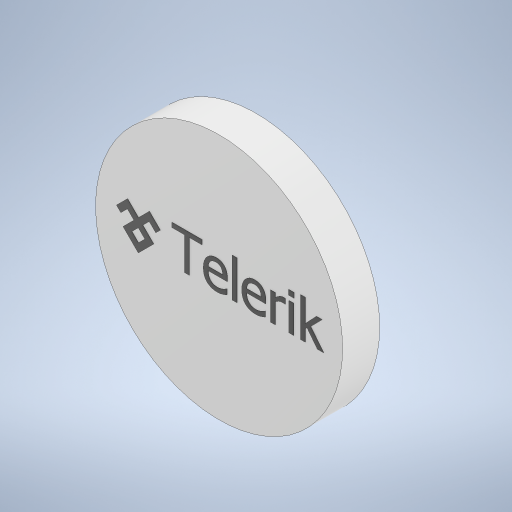
# Autodesk Inventor part: Logo Wheel
Saved by Autodesk Inventor 2023 (Build 270158000, 158)
## iProperties
Created: 2022-05-02
Part Number: Logo Wheel
Material: Phenolic Resin
Document SubType Name: Modeling
Designer: Devin
Density: 1.38 g/cm^3
Appearance: Smooth - White
Author: Devin
Autodesk Inventor part; units mm, degrees
ref_plane "YZ Plane" through (0, 0, 0) normal (1, 0, 0) x (0, 1, 0)
ref_plane "XZ Plane" through (0, 0, 0) normal (0, 1, 0) x (-1, 0, 0)
ref_plane "XY Plane" through (0, 0, 0) normal (0, 0, 1) x (1, 0, 0)
sketch "Sketch1" plane through (0, 0, 0) normal (0, 0, 1) x (1, 0, 0)
  circle A0 centre (0, 0) radius 10.16
  dimension "d0" = 20.32
  constraints: 1 centre point, 1 coincident
  measures "d0" diameter of A0
extrude "Extrusion1" add sketch "Sketch1" along normal blind 3.048
shell "Shell1" thickness 1.27 removed faces 1 at (6.5114, 0.3794, 0)
sketch "Sketch2" plane through (0, 0, 1.778) normal (0, 0, -1) x (-1, 0, 0)
  circle A0 centre (0, 0) radius 2.032
  circle A1 centre (0, 0) radius 0.635
  dimension "d4" = 4.064
  dimension "d5" = 1.27
  constraints: 2 centre point, 2 coincident
  measures "d4" diameter of A0
  measures "d5" diameter of A1
extrude "Extrusion2" add sketch "Sketch2" along normal blind 4.826
sketch "Sketch4" plane through (0, 0, 3.048) normal (0, 0, 1) x (1, 0, 0)
  line L0 (-3.849, 2.1267) -> (9.0262, 2.1267) construction
  line L1 (9.0262, 2.1267) -> (9.0262, -1.4869) construction
  line L2 (9.0262, -1.4869) -> (-3.849, -1.4869) construction
  line L3 (-3.849, -1.4869) -> (-3.849, 2.1267) construction
  line L4 (-8.4196, 0.9488) -> (-7.5216, 1.8468)
  line L5 (-7.5216, 1.8468) -> (-6.6236, 0.9488)
  line L6 (-6.6236, 0.9488) -> (-5.7256, 1.8468)
  line L7 (-5.7256, 1.8468) -> (-4.8275, 0.9488)
  line L8 (-8.0604, 0.5896) -> (-7.5216, 1.1284)
  line L9 (-7.5216, 1.1284) -> (-6.9828, 0.5896)
  line L10 (-6.2644, 0.5896) -> (-5.7256, 1.1284)
  line L11 (-5.7256, 1.1284) -> (-5.1867, 0.5896)
  line L12 (-8.4196, 0.9488) -> (-8.0604, 0.5896)
  line L13 (-5.1867, 0.5896) -> (-4.8275, 0.9488)
  line L14 (-6.9828, 0.5896) -> (-7.8808, -0.3084)
  line L15 (-7.8808, -0.3084) -> (-6.6236, -1.5657)
  line L16 (-6.6236, -1.5657) -> (-5.3663, -0.3084)
  line L17 (-5.3663, -0.3084) -> (-6.2644, 0.5896)
  line L18 (-6.6236, 0.2304) -> (-7.1624, -0.3084)
  line L19 (-7.1624, -0.3084) -> (-6.6236, -0.8473)
  line L20 (-6.6236, -0.8473) -> (-6.0848, -0.3084)
  line L21 (-6.0848, -0.3084) -> (-6.6236, 0.2304)
  line L22 (-2.8289, -1.0571) -> (-2.8289, 1.6302)
  line L23 (-2.8289, 1.6302) -> (-3.8514, 1.6302)
  line L24 (-3.8514, 1.6302) -> (-3.8514, 1.9909)
  line L25 (-3.8514, 1.9909) -> (-1.4012, 1.9909)
  line L26 (-1.4012, 1.9909) -> (-1.4012, 1.6302)
  line L27 (-1.4012, 1.6302) -> (-2.4238, 1.6302)
  line L28 (-2.4238, 1.6302) -> (-2.4238, -1.0571)
  line L29 (-2.4238, -1.0571) -> (-2.8289, -1.0571)
  spline S0 degree 2 poles (-0.1291, -1.109) (-0.6775, -1.109) (-1.2802, -0.494) (-1.2802, 0.0741) knots 0 0 0 1 2 2 2
  spline S1 degree 2 poles (-1.2802, 0.0741) (-1.2802, 0.6324) (-0.6948, 1.2943) (-0.223, 1.2943) knots 0 0 0 1 2 2 2
  spline S2 degree 2 poles (-0.223, 1.2943) (-0.0106, 1.2943) (0.3179, 1.1708) (0.439, 1.0399) knots 0 0 0 1 2 2 2
  spline S3 degree 2 poles (0.439, 1.0399) (0.5625, 0.909) (0.6934, 0.5311) (0.6934, 0.2569) knots 0 0 0 1 2 2 2
  line L30 (0.6934, 0.2569) -> (0.6934, 0.047)
  line L31 (0.6934, 0.047) -> (-0.8899, 0.047)
  spline S4 degree 2 poles (-0.8899, 0.047) (-0.8899, -0.3507) (-0.4897, -0.7731) (-0.1341, -0.7731) knots 0 0 0 1 2 2 2
  spline S5 degree 2 poles (-0.1341, -0.7731) (-0.0081, -0.7731) (0.2364, -0.7163) (0.3352, -0.6718) knots 0 0 0 1 2 2 2
  spline S6 degree 2 poles (0.3352, -0.6718) (0.439, -0.6224) (0.5822, -0.536) (0.6292, -0.4964) knots 0 0 0 1 2 2 2
  line L32 (0.6292, -0.4964) -> (0.6514, -0.4964)
  line L33 (0.6514, -0.4964) -> (0.6514, -0.9163)
  spline S7 degree 2 poles (0.6514, -0.9163) (0.5847, -0.9435) (0.3822, -1.0226) (0.3031, -1.0448) knots 0 0 0 1 2 2 2
  spline S8 degree 2 poles (0.3031, -1.0448) (0.192, -1.0769) (0.0092, -1.109) (-0.1291, -1.109) knots 0 0 0 1 2 2 2
  spline S9 degree 2 poles (0.3179, 0.3409) (0.313, 0.4965) (0.2488, 0.7237) (0.187, 0.8003) knots 0 0 0 1 2 2 2
  spline S10 degree 2 poles (0.187, 0.8003) (0.1203, 0.8868) (-0.0896, 0.9782) (-0.2452, 0.9782) knots 0 0 0 1 2 2 2
  spline S11 degree 2 poles (-0.2452, 0.9782) (-0.3984, 0.9782) (-0.6132, 0.8868) (-0.7022, 0.7979) knots 0 0 0 1 2 2 2
  spline S12 degree 2 poles (-0.7022, 0.7979) (-0.7886, 0.7065) (-0.8775, 0.4866) (-0.8899, 0.3409) knots 0 0 0 1 2 2 2
  line L34 (-0.8899, 0.3409) -> (0.3179, 0.3409)
  line L35 (1.4764, -1.0571) -> (1.0911, -1.0571)
  line L36 (1.0911, -1.0571) -> (1.0911, 2.1267)
  line L37 (1.0911, 2.1267) -> (1.4764, 2.1267)
  line L38 (1.4764, 2.1267) -> (1.4764, -1.0571)
  spline S13 degree 2 poles (3.035, -1.109) (2.4866, -1.109) (1.8839, -0.494) (1.8839, 0.0741) knots 0 0 0 1 2 2 2
  spline S14 degree 2 poles (1.8839, 0.0741) (1.8839, 0.6324) (2.4693, 1.2943) (2.9411, 1.2943) knots 0 0 0 1 2 2 2
  spline S15 degree 2 poles (2.9411, 1.2943) (3.1535, 1.2943) (3.482, 1.1708) (3.6031, 1.0399) knots 0 0 0 1 2 2 2
  spline S16 degree 2 poles (3.6031, 1.0399) (3.7266, 0.909) (3.8575, 0.5311) (3.8575, 0.2569) knots 0 0 0 1 2 2 2
  line L39 (3.8575, 0.2569) -> (3.8575, 0.047)
  line L40 (3.8575, 0.047) -> (2.2742, 0.047)
  spline S17 degree 2 poles (2.2742, 0.047) (2.2742, -0.3507) (2.6743, -0.7731) (3.03, -0.7731) knots 0 0 0 1 2 2 2
  spline S18 degree 2 poles (3.03, -0.7731) (3.156, -0.7731) (3.4005, -0.7163) (3.4993, -0.6718) knots 0 0 0 1 2 2 2
  spline S19 degree 2 poles (3.4993, -0.6718) (3.6031, -0.6224) (3.7463, -0.536) (3.7933, -0.4964) knots 0 0 0 1 2 2 2
  line L41 (3.7933, -0.4964) -> (3.8155, -0.4964)
  line L42 (3.8155, -0.4964) -> (3.8155, -0.9163)
  spline S20 degree 2 poles (3.8155, -0.9163) (3.7488, -0.9435) (3.5463, -1.0226) (3.4672, -1.0448) knots 0 0 0 1 2 2 2
  spline S21 degree 2 poles (3.4672, -1.0448) (3.3561, -1.0769) (3.1733, -1.109) (3.035, -1.109) knots 0 0 0 1 2 2 2
  spline S22 degree 2 poles (3.482, 0.3409) (3.4771, 0.4965) (3.4129, 0.7237) (3.3511, 0.8003) knots 0 0 0 1 2 2 2
  spline S23 degree 2 poles (3.3511, 0.8003) (3.2844, 0.8868) (3.0745, 0.9782) (2.9189, 0.9782) knots 0 0 0 1 2 2 2
  spline S24 degree 2 poles (2.9189, 0.9782) (2.7657, 0.9782) (2.5508, 0.8868) (2.4619, 0.7979) knots 0 0 0 1 2 2 2
  spline S25 degree 2 poles (2.4619, 0.7979) (2.3755, 0.7065) (2.2866, 0.4866) (2.2742, 0.3409) knots 0 0 0 1 2 2 2
  line L43 (2.2742, 0.3409) -> (3.482, 0.3409)
  line L44 (5.4605, 0.8176) -> (5.4408, 0.8176)
  spline S26 degree 2 poles (5.4408, 0.8176) (5.3963, 0.83) (5.3, 0.8349) (5.2333, 0.8349) knots 0 0 0 1 2 2 2
  spline S27 degree 2 poles (5.2333, 0.8349) (5.0777, 0.8349) (4.7714, 0.699) (4.6331, 0.5657) knots 0 0 0 1 2 2 2
  line L45 (4.6331, 0.5657) -> (4.6331, -1.0571)
  line L46 (4.6331, -1.0571) -> (4.2477, -1.0571)
  line L47 (4.2477, -1.0571) -> (4.2477, 1.2301)
  line L48 (4.2477, 1.2301) -> (4.6331, 1.2301)
  line L49 (4.6331, 1.2301) -> (4.6331, 0.8892)
  spline S28 degree 2 poles (4.6331, 0.8892) (4.843, 1.077) (5.1567, 1.2301) (5.3049, 1.2301) knots 0 0 0 1 2 2 2
  spline S29 degree 2 poles (5.3049, 1.2301) (5.3642, 1.2301) (5.4235, 1.2252) (5.4605, 1.2178) knots 0 0 0 1 2 2 2
  line L50 (5.4605, 1.2178) -> (5.4605, 0.8176)
  line L51 (6.1521, -1.0571) -> (5.7668, -1.0571)
  line L52 (5.7668, -1.0571) -> (5.7668, 1.2301)
  line L53 (5.7668, 1.2301) -> (6.1521, 1.2301)
  line L54 (6.1521, 1.2301) -> (6.1521, -1.0571)
  line L55 (6.1793, 1.6105) -> (5.7421, 1.6105)
  line L56 (5.7421, 1.6105) -> (5.7421, 2.0106)
  line L57 (5.7421, 2.0106) -> (6.1793, 2.0106)
  line L58 (6.1793, 2.0106) -> (6.1793, 1.6105)
  line L59 (8.6123, -1.0571) -> (8.1059, -1.0571)
  line L60 (8.1059, -1.0571) -> (7.2562, 0.047)
  line L61 (7.2562, 0.047) -> (7.1031, -0.1012)
  line L62 (7.1031, -0.1012) -> (7.1031, -1.0571)
  line L63 (7.1031, -1.0571) -> (6.7178, -1.0571)
  line L64 (6.7178, -1.0571) -> (6.7178, 2.1267)
  line L65 (6.7178, 2.1267) -> (7.1031, 2.1267)
  line L66 (7.1031, 2.1267) -> (7.1031, 0.2643)
  line L67 (7.1031, 0.2643) -> (8.0071, 1.2301)
  line L68 (8.0071, 1.2301) -> (8.4863, 1.2301)
  line L69 (8.4863, 1.2301) -> (7.5477, 0.2742)
  line L70 (7.5477, 0.2742) -> (8.6123, -1.0571)
  point P0 (0, 0)
  dimension "d12" = 1.27
  dimension "d13" = 1.27
  dimension "d14" = 1.27
  dimension "d15" = 1.27
  dimension "d16" = 0.508
  dimension "d17" = 1.27
  dimension "d18" = 0.508
  dimension "d19" = 0.5388
  dimension "d20" = 90
  dimension "d21" = 90
  dimension "d22" = 90
  dimension "d23" = 0.508
  dimension "d24" = 0.762
  dimension "d25" = 90
  dimension "d26" = 90
  dimension "d27" = 0.5388
  dimension "d28" = 90
  constraints: 36 end point, 6 perpendicular, 6 point on line, 5 other
  measures "d12" distance of L4.start L4.end
  measures "d13" distance of L4.end L5.end
  measures "d14" distance of L5.end L6.end
  measures "d15" distance of L6.end L7.end
  measures "d16" distance between parallel lines of L4 L8
  measures "d17" distance of L9.end L14.end
  measures "d18" distance between parallel lines of L14 L18
  measures "d19" horizontal distance of L20.end L21.end
  measures "d20" angle of L6 L5
  measures "d21" angle of L11 L13
  measures "d22" angle of L16 L17
  measures "d23" distance from line of L11 L7.end
  measures "d24" distance of L10.start L10.end
  measures "d25" angle of L21 L18
  measures "d26" angle of L12 L4
  measures "d27" horizontal distance of L18.start L18.end
  measures "d28" angle of L14 L9
emboss "Emboss1" sketch "Sketch4" operation add depth 0.0254 direction (0, 0, -1)
body "Solid1"
